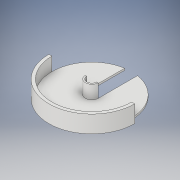
# Autodesk Inventor part: casept1
Saved by Autodesk Inventor 2017 (Build 210142000, 142)
## iProperties
Created: 2018-03-21
Part Number: casept1
Material: PC/ABS Plastic
Document SubType Name: Modeling
Designer: FablabGuest
Density: 0.357273 g/cm^3
Appearance: Smooth - White
Author: FablabGuest
Autodesk Inventor part; units mm, degrees
ref_plane "YZ Plane" through (0, 0, 0) normal (1, 0, 0) x (0, 1, 0)
ref_plane "XZ Plane" through (0, 0, 0) normal (0, 1, 0) x (-1, 0, 0)
ref_plane "XY Plane" through (0, 0, 0) normal (0, 0, 1) x (1, 0, 0)
sketch "Sketch1" plane through (0, 0, 0) normal (0, 1, 0) x (-1, 0, 0)
  circle A0 centre (0, 0) radius 70
  dimension "d0" = 140
  constraints: 1 centre point, 1 coincident
  measures "d0" diameter of A0
extrude "Extrusion1" add sketch "Sketch1" along normal blind 28
sketch "Sketch2" plane through (0, 28, 0) normal (0, 1, 0) x (1, 0, 0)
  circle A0 centre (0, 0) radius 8.25
  dimension "d3" = 16.5
  constraints: 1 centre point, 1 coincident
  measures "d3" diameter of A0
extrude "Extrusion2" cut sketch "Sketch2" against normal blind 280
sketch "Sketch3" plane through (0, 28, 0) normal (0, 1, 0) x (1, 0, 0)
  circle A0 centre (0, 0) radius 8.25 projected
  circle A1 centre (0, 0) radius 65
  circle A2 centre (0, 0) radius 10.5
  dimension "d6" = 130
  dimension "d7" = 21
  constraints: 2 centre point, 2 coincident
  measures "d6" diameter of A1
  measures "d7" diameter of A2
extrude "Extrusion3" cut sketch "Sketch3" against normal blind 22 contours A1
sketch "Sketch4" plane through (0, 6, 0) normal (0, 1, 0) x (1, 0, 0)
  line L0 (-77.4845, 0) -> (88.5537, 0)
  line L1 (88.5537, 0) -> (88.5537, 100.8261)
  line L2 (88.5537, 100.8261) -> (-77.4845, 100.8261)
  line L3 (-77.4845, 100.8261) -> (-77.4845, 0)
  point P0 (0, 0)
  constraints: 8 end point, 2 parallel, 1 horizontal, 1 perpendicular
extrude "Extrusion4" cut sketch "Sketch4" along normal blind 220
sketch "Sketch5" plane through (0, 0, 0) normal (0, -1, 0) x (1, 0, 0)
  circle A0 centre (0, 0) radius 8.25 projected
  circle A1 centre (0, 0) radius 70
  constraints: 1 centre point, 1 coincident
extrude "Extrusion5" cut sketch "Sketch5" against normal blind 3
sketch "Sketch6" plane through (0, 6, 0) normal (0, 1, 0) x (1, 0, 0)
  arc A0 (-65, 0) -> (65, 0) centre (0, 0) ccw projected
  line L0 (65, 0) -> (70, 0) projected
  arc A1 (70, 0) -> (-70, 0) centre (0, 0) ccw projected
  line L1 (-70, 0) -> (-65, 0) projected
  arc A2 (-10.5, 0) -> (10.5, 0) centre (0, 0) ccw projected
  line L2 (-10.5, 0) -> (-8.25, 0) projected
  arc A3 (8.25, 0) -> (-8.25, 0) centre (0, 0) ccw projected
  line L3 (8.25, 0) -> (10.5, 0) projected
  circle A4 centre (0, 0) radius 8.25 projected
  arc A5 (65, 0) -> (-65, 0) centre (0, 0) ccw
  line L4 (-65, 0) -> (-70, 0)
  line L5 (65, 0) -> (70, 0)
  arc A6 (70, 0) -> (-70, 0) centre (0, 0) ccw projected
  arc A7 (70, 0) -> (70, 0) centre (0, 0) ccw
  constraints: 4 end point, 3 point on circle, 2 coincident, 2 horizontal, 1 centre point, 1 horizontal alignment, 3 other
extrude "Extrusion6" cut sketch "Sketch6" against normal blind 3 contours L1 A1 L0 A5
sketch "Sketch7" plane through (0, 3, 0) normal (0, -1, 0) x (1, 0, 0)
  point P0 (0, 0)
sketch "Sketch8" plane through (0, 3, 0) normal (0, -1, 0) x (1, 0, 0)
  arc A0 (65, 0) -> (-65, 0) centre (0, 0) ccw projected
  arc A1 (70, 0) -> (-70, 0) centre (0, 0) ccw projected
  arc A2 (70, 0) -> (-70, 0) centre (0, 0) ccw
  arc A3 (65, 0) -> (-65, 0) centre (0, 0) ccw
  line L0 (65, 0) -> (70, 0) projected
  line L1 (70, 0) -> (65, 0)
  line L2 (-65, 0) -> (-70, 0) projected
  line L3 (-65, 0) -> (-70, 0)
  constraints: 4 end point, 4 point on circle, 2 centre point, 2 coincident, 2 horizontal
extrude "Extrusion7" add sketch "Sketch8" along normal blind 3
sketch "Sketch9" plane through (0, 28, 0) normal (0, 1, 0) x (1, 0, 0)
  line L0 (10.5, 0) -> (-10.497, 0)
  line L1 (-10.497, 0) -> (-10.497, 68.6752)
  line L2 (-10.497, 68.6752) -> (10.5, 68.6752)
  line L3 (10.5, 68.6752) -> (10.5, 0)
  point P0 (0, 0)
  constraints: 8 end point, 2 parallel, 1 horizontal, 1 perpendicular
extrude "Extrusion8" cut sketch "Sketch9" against normal blind 30
body "Solid1"
